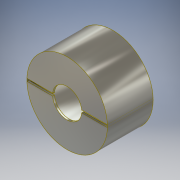
# Autodesk Inventor part: dis1
Saved by Autodesk Inventor 2018 (Build 220112000, 112)
## iProperties
Created: 2019-04-16
Part Number: dis1
Material: Generic
Document SubType Name: Modeling
Designer: This kid
Density: 1 g/cm^3
Appearance: Silver
Author: This kid
Autodesk Inventor part; units mm, degrees
ref_plane "YZ Plane" through (0, 0, 0) normal (1, 0, 0) x (0, 1, 0)
ref_plane "XZ Plane" through (0, 0, 0) normal (0, 1, 0) x (-1, 0, 0)
ref_plane "XY Plane" through (0, 0, 0) normal (0, 0, 1) x (1, 0, 0)
sketch "Sketch1" plane through (0, 0, 0) normal (0, 0, 1) x (1, 0, 0)
  circle A0 centre (0, 0) radius 8.255
  circle A1 centre (0, 0) radius 2.9845
  line L0 (-8.2498, 0.2936) -> (-2.9768, 0.2936)
  line L1 (-2.9768, 0.2936) -> (-2.9768, -0.2144)
  line L2 (-2.9768, -0.2144) -> (-8.2498, -0.2144)
  line L3 (-8.1951, 0.2936) -> (-8.1951, -0.2144)
  line L4 (0, 8.255) -> (0, -8.255) construction
  line L5 (8.2498, 0.2936) -> (2.9768, 0.2936)
  line L6 (2.9768, 0.2936) -> (2.9768, -0.2144)
  line L7 (2.9768, -0.2144) -> (8.2498, -0.2144)
  line L8 (8.1951, 0.2936) -> (8.1951, -0.2144)
  dimension "d13" = 5.969
  dimension "d0" = 16.51
  dimension "d14" = 0.508
  constraints: 18 end point, 6 symmetric about line, 4 point on line, 3 point on circle, 2 coincident, 2 perpendicular, 1 centre point, 1 horizontal, 1 parallel, 1 vertical, 3 other
  measures "d0" diameter of A0
  measures "d14" distance of L0.end L1.end
extrude "Extrusion1" add sketch "Sketch1" along normal blind 9.3726
shell "Shell1" thickness 0.381 removed faces 1 at (-0.9758, 3.8899, 0)
extrude "Extrusion3" cut sketch "Sketch1" along normal blind 17.526 contours L0 L1 A1 L2 L3 | L1 A1
extrude "Extrusion4" cut sketch "Sketch1" along normal blind 17.526 contours L6 A1 L1 | A1 L6 | L1 A1
extrude "Extrusion5" cut sketch "Sketch1" along normal blind 17.526 contours L8 L7 A1 L6 L5 | A1 L6
body "Solid1"
